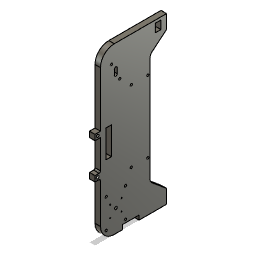
Конвеер Сторона v27 (Autodesk Fusion 360 design; units mm, degrees)
Autodesk Fusion 360 part; units mm, degrees
sketch "Sketch1" plane through (0, 0, 0) normal (1, 0, 0) x (0, 1, 0)
  line L0 (-300, 0) -> (-300, 75)
  line L1 (-275, 100) -> (-25, 100)
  line L2 (0, 75) -> (0, 0)
  arc A0 (-275, 100) -> (-300, 75) centre (-275, 75) ccw
  arc A1 (0, 75) -> (-25, 100) centre (-25, 75) ccw
  line L3 (-300, 0) -> (-300, 25)
  circle A2 centre (-20, 85) radius 5
  circle A3 centre (-280, 85) radius 5
  line L4 (-300, 60) -> (-292, 60)
  line L5 (-292, 60) -> (-292, 30)
  line L6 (-292, 30) -> (-300, 30)
  line L7 (-300, 30) -> (-300, 60)
  line L8 (0, 30) -> (-8, 30)
  line L9 (-8, 30) -> (-8, 60)
  line L10 (-8, 60) -> (0, 60)
  line L11 (0, 60) -> (0, 30)
  line L12 (-275, -20) -> (-300, -20)
  line L13 (-300, -20) -> (-300, 0)
  line L14 (-25, -20) -> (0, -20)
  line L15 (0, -20) -> (0, 0)
  line L16 (-275, -20) -> (-252.9985, 6.4018)
  line L17 (-245.3163, 10) -> (-54.6837, 10)
  line L18 (-47.0015, 6.4018) -> (-25, -20)
  arc A4 (-245.3163, 10) -> (-252.9985, 6.4018) centre (-245.3163, 0) ccw
  arc A5 (-47.0015, 6.4018) -> (-54.6837, 10) centre (-54.6837, 0) ccw
  point P0 (0, 100)
  dimension "d1" = 300
  dimension "d2" = 100
  dimension "d79" = 25
  dimension "d80" = 25
  dimension "d87" = 10
  dimension "d88" = 8
  dimension "d89" = 30
  dimension "d90" = 8
  dimension "d91" = 30
  dimension "d144" = 40
  dimension "d145" = 10
  dimension "d146" = 10
  dimension "d147" = 20
  dimension "d148" = 20
  dimension "d150" = 40
  dimension "d188" = 20
  dimension "d190" = 20
  dimension "d191" = 10
  dimension "d192" = 10
  dimension "d193" = 90
  dimension "d194" = 34.3675
  dimension "d195" = 54.6837
  dimension "d196" = 34.3675
  dimension "d197" = 54.6837
  dimension "d198" = 25
  dimension "d199" = 260
  constraint vertical L0
  constraint horizontal L1
  constraint vertical L2
  constraint coincident L2.end L15.end
  constraint tangent L1 A0
  constraint tangent L0 A0
  constraint coincident P0 L2
  constraint coincident P0 L1
  constraint tangent L2 A1
  constraint tangent L1 A1
  constraint vertical L3
  constraint coincident L0 L3.end
  constraint horizontal L4
  constraint vertical L5
  constraint horizontal L6
  constraint vertical L7
  constraint coincident L0 L4.start
  constraint horizontal L8
  constraint vertical L9
  constraint horizontal L10
  constraint vertical L11
  constraint coincident L2 L8.start
  constraint horizontal L12
  constraint vertical L13
  constraint horizontal L14
  constraint vertical L15
  constraint tangent L16 A4
  constraint tangent L17 A4
  constraint tangent L18 A5
  constraint tangent L17 A5
  measures "d1" distance of L2.end L0.start
  measures "d2" distance of L2.end P0
  measures "d79" radius of A0
  measures "d80" radius of A1
  measures "d87" diameter of A3
  measures "d88" distance of L4.start L4.end
  measures "d89" distance of L4.start L6.end
  measures "d90" distance of L8.start L8.end
  measures "d91" distance of L8.start L10.end
  measures "d144" distance of L1 L10
  measures "d145" vertical distance of A1.centre A2.centre
  measures "d146" diameter of A2
  measures "d147" distance of L2 A2.centre
  measures "d148" distance of L0 A3.centre
  measures "d150" distance of L1 L4
  measures "d188" distance of L0.start L12.end
  measures "d190" distance of L2.end L14.end
  measures "d191" radius of A4
  measures "d192" radius of A5
  measures "d193" distance of L1 L17
  measures "d194" distance of L14.start L18.start
  measures "d195" distance of L2 A5.centre
  measures "d196" distance of L12.start L16.end
  measures "d197" distance of L0 A4.centre
  measures "d198" distance of L12.start L12.end
  measures "d199" distance of A2.centre A3.centre
extrude "Extrude1" add sketch "Sketch1" along normal blind 10 contours L0 L1 L2 A0 A1 L3 L4 L5 L6 L8 L9 L10 L12 L13 L14 L15 L16 L17 L18 A4 A5 | A2 | A3
sketch "Sketch2" plane through (10, 0, 0) normal (1, 0, 0) x (0, 1, 0)
  arc A0 (0, 75) -> (-25, 100) centre (-25, 75) ccw
  line L0 (-25, 100) -> (-275, 100)
  arc A1 (-275, 100) -> (-300, 75) centre (-275, 75) ccw
  line L1 (-300, 75) -> (-300, 60)
  line L2 (0, 60) -> (0, 75)
  line L3 (-8, 30) -> (-8, 60)
  line L4 (-8, 60) -> (0, 60)
  line L5 (-300, 60) -> (-292, 60)
  line L6 (-292, 60) -> (-292, 30)
  line L7 (-292, 30) -> (-300, 30)
  line L8 (-300, 30) -> (-300, -20)
  line L9 (-300, -20) -> (-275, -20)
  line L10 (-275, -20) -> (-252.9985, 6.4018)
  arc A2 (-245.3163, 10) -> (-252.9985, 6.4018) centre (-245.3163, 0) ccw
  line L11 (-245.3163, 10) -> (-54.6837, 10)
  arc A3 (-47.0015, 6.4018) -> (-54.6837, 10) centre (-54.6837, 0) ccw
  line L12 (-47.0015, 6.4018) -> (-25, -20)
  line L13 (-25, -20) -> (0, -20)
  line L14 (0, -20) -> (0, 30)
  line L15 (0, 30) -> (-8, 30)
sketch "Sketch7" plane through (10, 0, 0) normal (1, 0, 0) x (0, 1, 0)
sketch "Sketch8" plane through (10, 0, 0) normal (1, 0, 0) x (0, 1, 0)
sketch "Sketch10" plane through (10, 0, 0) normal (1, 0, 0) x (0, 1, 0)
  line L0 (0, 60) -> (0, 75)
  arc A0 (0, 75) -> (-25, 100) centre (-25, 75) ccw
  line L1 (-25, 100) -> (-275, 100)
  arc A1 (-275, 100) -> (-300, 75) centre (-275, 75) ccw
  line L2 (-300, 75) -> (-300, 60)
  circle A2 centre (-25, 85) radius 5
  circle A3 centre (-275, 85) radius 5
  line L3 (-8, 30) -> (-8, 60)
  line L4 (-8, 60) -> (0, 60)
  line L5 (-300, 60) -> (-292, 60)
  line L6 (-292, 60) -> (-292, 30)
  line L7 (-292, 30) -> (-300, 30)
  line L8 (-300, 30) -> (-300, -20)
  line L9 (-300, -20) -> (-275, -20)
  line L10 (-275, -20) -> (-252.9985, 6.4018)
  arc A4 (-245.3163, 10) -> (-252.9985, 6.4018) centre (-245.3163, 0) ccw
  line L11 (-245.3163, 10) -> (-54.6837, 10)
  arc A5 (-47.0015, 6.4018) -> (-54.6837, 10) centre (-54.6837, 0) ccw
  line L12 (-47.0015, 6.4018) -> (-25, -20)
  line L13 (-25, -20) -> (0, -20)
  line L14 (0, -20) -> (0, 30)
  line L15 (0, 30) -> (-8, 30)
  point P0 (-80, 44)
  dimension "d96" = 10
  dimension "d98" = 10
  dimension "d260" = 25
  dimension "d261" = 25
  dimension "d262" = 25
  dimension "d263" = 25
  measures "d96" diameter of A2
  measures "d98" diameter of A3
  measures "d260" distance of L2 A3.centre
  measures "d261" distance of L0 A2.centre
  measures "d262" distance of A2.centre L4
  measures "d263" distance of A3.centre L5
extrude "Extrude11" cut sketch "Sketch10" against normal blind 100 contours A2 | A3
sketch "Sketch11" plane through (10, 0, 0) normal (1, 0, 0) x (0, 1, 0)
  circle A0 centre (-275, 85) radius 5
  circle A1 centre (-25, 85) radius 5
  line L0 (0, 60) -> (0, 75)
  arc A2 (0, 75) -> (-25, 100) centre (-25, 75) ccw
  line L1 (-25, 100) -> (-275, 100)
  arc A3 (-275, 100) -> (-300, 75) centre (-275, 75) ccw
  line L2 (-300, 75) -> (-300, 60)
  line L3 (-175, 90) -> (-175, 80)
  line L4 (-175, 80) -> (-125, 80)
  line L5 (-175, 80) -> (-125, 80)
  line L6 (-175, 90) -> (-175, 80)
  line L7 (-125, 80) -> (-125, 90)
  line L8 (-125, 90) -> (-175, 90)
  line L9 (-8, 30) -> (-8, 60)
  line L10 (-8, 60) -> (0, 60)
  line L11 (-300, 60) -> (-292, 60)
  line L12 (-292, 60) -> (-292, 30)
  line L13 (-292, 30) -> (-300, 30)
  line L14 (-300, 30) -> (-300, -20)
  line L15 (-300, -20) -> (-275, -20)
  line L16 (-275, -20) -> (-252.9985, 6.4018)
  arc A4 (-245.3163, 10) -> (-252.9985, 6.4018) centre (-245.3163, 0) ccw
  line L17 (-245.3163, 10) -> (-54.6837, 10)
  arc A5 (-47.0015, 6.4018) -> (-54.6837, 10) centre (-54.6837, 0) ccw
  line L18 (-47.0015, 6.4018) -> (-25, -20)
  line L19 (-25, -20) -> (0, -20)
  line L20 (0, -20) -> (0, 30)
  line L21 (0, 30) -> (-8, 30)
  dimension "d174" = 125
  dimension "d175" = 50
  dimension "d176" = 10
  dimension "d259" = 10
  constraint vertical L3
  constraint horizontal L4
  constraint horizontal L5
  constraint vertical L6
  constraint perpendicular L5 L7
  constraint perpendicular L6 L8
  measures "d174" distance of L2 L6
  measures "d175" distance of L3.start L7.end
  measures "d176" distance of L5 L8
  measures "d259" distance of L1 L8
sketch "Sketch12" plane through (10, 0, 0) normal (1, 0, 0) x (0, 1, 0)
  circle A0 centre (-275, 85) radius 5
  circle A1 centre (-25, 85) radius 5
  line L0 (0, 60) -> (0, 75)
  arc A2 (0, 75) -> (-25, 100) centre (-25, 75) ccw
  line L1 (-25, 100) -> (-275, 100)
  arc A3 (-275, 100) -> (-300, 75) centre (-275, 75) ccw
  line L2 (-300, 75) -> (-300, 60)
  line L3 (-275, 85) -> (-260, 85)
  line L4 (-260, 85) -> (-260, 72)
  circle A4 centre (-40, 72) radius 2.5
  circle A5 centre (-260, 72) radius 2.5
  circle A6 centre (-275, 85) radius 2.5
  circle A7 centre (-25, 85) radius 2.5
  line L5 (-8, 30) -> (-8, 60)
  line L6 (-8, 60) -> (0, 60)
  line L7 (-300, 60) -> (-292, 60)
  line L8 (-292, 60) -> (-292, 30)
  line L9 (-292, 30) -> (-300, 30)
  line L10 (-300, 30) -> (-300, -20)
  line L11 (-300, -20) -> (-275, -20)
  line L12 (-275, -20) -> (-252.9985, 6.4018)
  arc A8 (-245.3163, 10) -> (-252.9985, 6.4018) centre (-245.3163, 0) ccw
  line L13 (-245.3163, 10) -> (-54.6837, 10)
  arc A9 (-47.0015, 6.4018) -> (-54.6837, 10) centre (-54.6837, 0) ccw
  line L14 (-47.0015, 6.4018) -> (-25, -20)
  line L15 (-25, -20) -> (0, -20)
  line L16 (0, -20) -> (0, 30)
  line L17 (0, 30) -> (-8, 30)
  dimension "d104" = 13
  dimension "d106" = 5
  dimension "d107" = 5
  dimension "d163" = 5
  dimension "d164" = 5
  dimension "d170" = 15
  dimension "d254" = 28
  dimension "d256" = 40
  dimension "d257" = 10
  dimension "d258" = 15
  constraint coincident A0.centre L3.start
  constraint horizontal L3
  constraint perpendicular L3 L4
  constraint coincident L4.end A5.centre
  constraint concentric A0 A6
  measures "d104" distance of L3.end L4.end
  measures "d106" diameter of A4
  measures "d107" diameter of A5
  measures "d163" diameter of A7
  measures "d164" diameter of A6
  measures "d170" distance of A0.centre L3.end
  measures "d254" distance of L1 A4.centre
  measures "d256" distance of L0 A4.centre
  measures "d257" distance of A2.centre A1.centre
  measures "d258" distance of A2.end A1.centre
extrude "Extrude13" cut sketch "Sketch12" against normal blind 40 contours A4 | A5
extrude "Extrude14" add sketch "Sketch12" against normal blind 10 contours A0 | A1 | A6 | A7
sketch "Sketch13" plane through (0, 0, 100) normal (0, 0, 1) x (-1, 0, 0)
  line L0 (0, 25) -> (0, 275)
  line L1 (0, 275) -> (-10, 275)
  line L2 (-10, 275) -> (-10, 25)
  line L3 (-10, 25) -> (0, 25)
  line L4 (0, 200) -> (-10, 200)
  line L5 (-10, 200) -> (-10, 190)
  line L6 (-10, 190) -> (0, 190)
  line L7 (0, 190) -> (0, 200)
  dimension "d251" = 10
  dimension "d253" = 75
  constraint horizontal L4
  constraint vertical L5
  constraint horizontal L6
  constraint vertical L7
  constraint coincident L2 L5.end
  constraint coincident L0 L4.start
  measures "d251" distance of L4 L6
  measures "d253" distance of L1 L4
extrude "Extrude15" add sketch "Sketch13" along normal blind 10 contours L0 L2 L4 L5 L6 L7
sketch "Sketch14" plane through (10, 0, 0) normal (1, 0, 0) x (0, 1, 0)
  circle A0 centre (-40, 72) radius 2.5
  circle A1 centre (-260, 72) radius 2.5
  line L0 (0, 60) -> (0, 75)
  arc A2 (0, 75) -> (-25, 100) centre (-25, 75) ccw
  line L1 (-25, 100) -> (-190, 100)
  line L2 (-190, 110) -> (-200, 110)
  arc A3 (-275, 100) -> (-300, 75) centre (-275, 75) ccw
  line L3 (-300, 75) -> (-300, 60)
  line L4 (-190, 100) -> (-190, 110)
  circle A4 centre (-195, 105.2223) radius 1.5
  circle A5 centre (-195, 105.2223) radius 2.5
  line L5 (-190, 100) -> (-190, 110)
  line L6 (-200, 110) -> (-200, 100)
  line L7 (-200, 100) -> (-275, 100)
  line L8 (-8, 30) -> (-8, 60)
  line L9 (-8, 60) -> (0, 60)
  line L10 (-300, 60) -> (-292, 60)
  line L11 (-292, 60) -> (-292, 30)
  line L12 (-292, 30) -> (-300, 30)
  line L13 (-300, 30) -> (-300, -20)
  line L14 (-300, -20) -> (-275, -20)
  line L15 (-275, -20) -> (-252.9985, 6.4018)
  arc A6 (-245.3163, 10) -> (-252.9985, 6.4018) centre (-245.3163, 0) ccw
  line L16 (-245.3163, 10) -> (-54.6837, 10)
  arc A7 (-47.0015, 6.4018) -> (-54.6837, 10) centre (-54.6837, 0) ccw
  line L17 (-47.0015, 6.4018) -> (-25, -20)
  line L18 (-25, -20) -> (0, -20)
  line L19 (0, -20) -> (0, 30)
  line L20 (0, 30) -> (-8, 30)
  dimension "d116" = 3
  dimension "d117" = 5
  dimension "d249" = 5
  dimension "d250" = 4.7777
  constraint coincident L2.start L4.end
  constraint perpendicular L2 L4
  constraint concentric A4 A5
  measures "d116" diameter of A4
  measures "d117" diameter of A5
  measures "d249" distance of A4.centre L6
  measures "d250" distance of L2 A4.centre
extrude "Extrude16" cut sketch "Sketch14" against normal blind 13 contours A4 | A5
thread "Thread6" "ISO Metric profile 5.0 M5x0.8 6H" major diameter 5.12 minor diameter 4.234 pitch 0.8 angle 60 resizes the face on face at (6.6667, -194.2038, 107.5921)
sketch "Sketch15" plane through (10, 0, 0) normal (1, 0, 0) x (0, 1, 0)
  circle A0 centre (-195, 105.2223) radius 2.117
  circle A1 centre (-40, 72) radius 2.5
  circle A2 centre (-260, 72) radius 2.5
  line L0 (0, 60) -> (0, 75)
  arc A3 (0, 75) -> (-25, 100) centre (-25, 75) ccw
  line L1 (-25, 100) -> (-190, 100)
  line L2 (-190, 110) -> (-200, 110)
  arc A4 (-275, 100) -> (-300, 75) centre (-275, 75) ccw
  line L3 (-300, 75) -> (-300, 60)
  circle A5 centre (-195, 105.2223) radius 3
  line L4 (-190, 100) -> (-190, 110)
  line L5 (-200, 110) -> (-200, 100)
  line L6 (-200, 100) -> (-275, 100)
  line L7 (-8, 30) -> (-8, 60)
  line L8 (-8, 60) -> (0, 60)
  line L9 (-300, 60) -> (-292, 60)
  line L10 (-292, 60) -> (-292, 30)
  line L11 (-292, 30) -> (-300, 30)
  line L12 (-300, 30) -> (-300, -20)
  line L13 (-300, -20) -> (-275, -20)
  line L14 (-275, -20) -> (-252.9985, 6.4018)
  arc A6 (-245.3163, 10) -> (-252.9985, 6.4018) centre (-245.3163, 0) ccw
  line L15 (-245.3163, 10) -> (-54.6837, 10)
  arc A7 (-47.0015, 6.4018) -> (-54.6837, 10) centre (-54.6837, 0) ccw
  line L16 (-47.0015, 6.4018) -> (-25, -20)
  line L17 (-25, -20) -> (0, -20)
  line L18 (0, -20) -> (0, 30)
  line L19 (0, 30) -> (-8, 30)
  dimension "d120" = 6
  constraint concentric A0 A5
  measures "d120" diameter of A5
extrude "Extrude17" cut sketch "Sketch15" against normal blind 16.5 contours A5
thread "Thread7" "ISO Metric profile 6.0 M6x1 6H" major diameter 6.147 minor diameter 5.035 pitch 1 angle 60 resizes the face on face at (6.6667, -192.9053, 107.3699)
fillet "Fillet2" radius 2.5 2 edges at (5, -200, 100) (5, -190, 100)
sketch "Sketch16" plane through (10, 0, 0) normal (1, 0, 0) x (0, 1, 0)
  line L0 (-270.5, 61.5) -> (-249.5, 61.5)
  line L1 (-249.5, 61.5) -> (-249.5, 82.5)
  line L2 (-249.5, 82.5) -> (-270.5, 82.5)
  line L3 (-270.5, 82.5) -> (-270.5, 61.5)
  line L4 (-270.5, 61.5) -> (-249.5, 82.5) construction
  line L5 (-249.5, 61.5) -> (-270.5, 82.5) construction
  circle A0 centre (-270.5, 82.5) radius 1
  circle A1 centre (-249.5, 82.5) radius 1
  circle A2 centre (-249.5, 61.5) radius 1
  circle A3 centre (-270.5, 61.5) radius 1
  line L6 (-290, 93) -> (-230, 93)
  line L7 (-230, 93) -> (-230, 51)
  line L8 (-230, 51) -> (-290, 51)
  line L9 (-290, 51) -> (-290, 93)
  line L10 (-290, 93) -> (-230, 51) construction
  line L11 (-230, 93) -> (-290, 51) construction
  line L12 (-260, 72) -> (-245.6634, 92.4808)
  line L13 (-260, 72) -> (-260, 89.5)
  line L14 (-260, 89.5) -> (-233.5, 89.5)
  line L15 (-233.5, 89.5) -> (-286.5, 89.5)
  line L16 (-260, 72) -> (-260, 54.5)
  circle A4 centre (-286.5, 89.5) radius 2
  circle A5 centre (-233.5, 89.5) radius 2
  line L17 (-260, 54.5) -> (-286.5, 54.5)
  line L18 (-286.5, 54.5) -> (-233.5, 54.5)
  circle A6 centre (-286.5, 54.5) radius 2
  circle A7 centre (-233.5, 54.5) radius 2
  point P0 (-260, 72)
  point P1 (-260, 72)
  point P2 (-260, 72)
  dimension "d127" = 21
  dimension "d128" = 21
  dimension "d129" = 2
  dimension "d130" = 2
  dimension "d131" = 2
  dimension "d132" = 2
  dimension "d133" = 60
  dimension "d134" = 42
  dimension "d135" = 25
  dimension "d165" = 17.5
  dimension "d166" = 26.5
  dimension "d167" = 53
  dimension "d168" = 17.5
  dimension "d179" = 4
  dimension "d180" = 4
  dimension "d181" = 53
  dimension "d182" = 4
  dimension "d183" = 4
  dimension "d184" = 26.5
  constraint horizontal L0
  constraint perpendicular L0 L1
  constraint parallel L0 L2
  constraint parallel L1 L3
  constraint coincident L4 P2
  constraint coincident L5 P2
  constraint coincident L2.end L3.start
  constraint coincident L1.end L2.start
  constraint coincident L0.end L1.start
  constraint coincident L0.start L3.end
  constraint horizontal L6
  constraint perpendicular L6 L7
  constraint parallel L6 L8
  constraint parallel L7 L9
  constraint coincident L10 P2
  constraint coincident L11 P2
  constraint coincident P2 P1
  constraint perpendicular L10 L12
  constraint perpendicular L2 L13
  constraint perpendicular L13 L14
  constraint perpendicular L13 L15
  constraint perpendicular L0 L16
  constraint coincident L15.end A4.centre
  constraint coincident L14.end L15.start
  constraint perpendicular L16 L17
  constraint perpendicular L16 L18
  constraint coincident L17.end L18.start
  constraint coincident L18.end A7.centre
  measures "d127" distance of L1.end L2.end
  measures "d128" distance of L0.end L1.end
  measures "d129" diameter of A0
  measures "d130" diameter of A1
  measures "d131" diameter of A2
  measures "d132" diameter of A3
  measures "d133" distance of L7.end L8.end
  measures "d134" distance of L6.end L7.end
  measures "d135" distance of P2 L12.end
  measures "d165" distance of P2 L13.end
  measures "d166" distance of L13.end L14.end
  measures "d167" distance of L14.end L15.end
  measures "d168" distance of P2 L16.end
  measures "d179" diameter of A4
  measures "d180" diameter of A5
  measures "d181" distance of L17.end L18.end
  measures "d182" diameter of A6
  measures "d183" diameter of A7
  measures "d184" distance of L16 L17.end
extrude "Extrude23" cut sketch "Sketch11" against normal blind 60 contours L3 L4 L5 L6 L7 L8
extrude "Extrude19" cut sketch "Sketch16" against normal blind 45 contours L0 L3 A3 | L0 L3 A3 | L2 L3 A0 | L2 L3 A0 | L0 L1 A2 | L0 L1 A2 | L1 L2 A1 | L1 L2 A1 | A4 | A5 | A6 | A7
sketch "Sketch18" plane through (10, 0, 0) normal (1, 0, 0) x (0, 1, 0)
  line L0 (-20, -9.7401) -> (-5, -9.7401)
  line L1 (-5, -9.7401) -> (-5, 0.2599)
  line L2 (-5, 0.2599) -> (-20, 0.2599)
  line L3 (-20, 0.2599) -> (-20, -9.7401)
  dimension "d155" = 10
  dimension "d200" = 15
  dimension "d247" = 5
  dimension "d248" = 0.2599
  constraint horizontal L0
  constraint vertical L1
  constraint horizontal L2
  constraint vertical L3
  measures "d155" distance of L0.end L1.end
  measures "d200" distance of L1.end L2.end
  measures "d247" distance of origin L1
  measures "d248" distance of origin L2
extrude "Extrude21" cut sketch "Sketch18" against normal blind 41
sketch "Sketch19" plane through (10, 0, 0) normal (1, 0, 0) x (0, 1, 0)
  line L0 (-135, 100) -> (-125, 100)
  line L1 (-125, 100) -> (-125, 110)
  line L2 (-125, 110) -> (-135, 110)
  line L3 (-135, 110) -> (-135, 100)
  circle A0 centre (-130, 105) radius 2.5
  dimension "d156" = 10
  dimension "d157" = 10
  dimension "d158" = 5
  dimension "d243" = 5
  dimension "d244" = 5
  dimension "d245" = 125
  dimension "d246" = 110
  constraint horizontal L0
  constraint vertical L1
  constraint horizontal L2
  constraint vertical L3
  measures "d156" distance of L1 L3
  measures "d157" distance of L0 L2
  measures "d158" diameter of A0
  measures "d243" distance of L0 A0.centre
  measures "d244" distance of L1 A0.centre
  measures "d245" distance of origin L1
  measures "d246" distance of origin L2
extrude "Extrude22" add sketch "Sketch19" against normal blind 10
sketch "Sketch20" plane through (10, 0, 0) normal (1, 0, 0) x (0, 1, 0)
  circle A0 centre (-130, 105) radius 2.5
  line L0 (-5, -9.7401) -> (-20, -9.7401)
  line L1 (-20, -9.7401) -> (-20, 0.2599)
  line L2 (-20, 0.2599) -> (-5, 0.2599)
  line L3 (-5, 0.2599) -> (-5, -9.7401)
  circle A1 centre (-233.5, 54.5) radius 2
  circle A2 centre (-249.5, 82.5) radius 1
  circle A3 centre (-249.5, 61.5) radius 1
  circle A4 centre (-286.5, 54.5) radius 2
  circle A5 centre (-233.5, 89.5) radius 2
  circle A6 centre (-270.5, 82.5) radius 1
  circle A7 centre (-270.5, 61.5) radius 1
  circle A8 centre (-286.5, 89.5) radius 2
  line L4 (-175, 80) -> (-175, 90)
  line L5 (-175, 90) -> (-125, 90)
  line L6 (-125, 90) -> (-125, 80)
  line L7 (-125, 80) -> (-175, 80)
  circle A9 centre (-195, 105.2223) radius 2.5175
  circle A10 centre (-40, 72) radius 2.5
  circle A11 centre (-260, 72) radius 2.5
  line L8 (0, 60) -> (0, 75)
  arc A12 (0, 75) -> (-25, 100) centre (-25, 75) ccw
  line L9 (-25, 100) -> (-125, 100)
  line L10 (-125, 100) -> (-125, 110)
  line L11 (-125, 110) -> (-135, 110)
  line L12 (-135, 110) -> (-135, 100)
  arc A13 (-190, 102.5) -> (-187.5, 100) centre (-187.5, 102.5) ccw
  line L13 (-190, 102.5) -> (-190, 110)
  line L14 (-190, 110) -> (-200, 110)
  line L15 (-200, 110) -> (-200, 102.5)
  arc A14 (-202.5, 100) -> (-200, 102.5) centre (-202.5, 102.5) ccw
  line L16 (-202.5, 100) -> (-275, 100)
  arc A15 (-275, 100) -> (-300, 75) centre (-275, 75) ccw
  line L17 (-300, 75) -> (-300, 60)
  line L18 (-40, 72) -> (-50, 72)
  line L19 (-50, 74.5) -> (-40, 74.5)
  line L20 (-40, 69.5) -> (-50, 69.5)
  arc A16 (-50, 74.5) -> (-50, 69.5) centre (-50, 72) ccw
  line L21 (-300, 60) -> (-292, 60)
  line L22 (-292, 60) -> (-292, 30)
  line L23 (-292, 30) -> (-300, 30)
  line L24 (-300, 30) -> (-300, -20)
  line L25 (-300, -20) -> (-275, -20)
  line L26 (-275, -20) -> (-252.9985, 6.4018)
  arc A17 (-245.3163, 10) -> (-252.9985, 6.4018) centre (-245.3163, 0) ccw
  line L27 (-245.3163, 10) -> (-54.6837, 10)
  arc A18 (-47.0015, 6.4018) -> (-54.6837, 10) centre (-54.6837, 0) ccw
  line L28 (-47.0015, 6.4018) -> (-25, -20)
  line L29 (-25, -20) -> (0, -20)
  line L30 (-8, 30) -> (-8, 60)
  line L31 (-8, 60) -> (0, 60)
  line L32 (-135, 100) -> (-187.5, 100)
  line L33 (0, -20) -> (0, 30)
  line L34 (0, 30) -> (-8, 30)
  dimension "d185" = 5
  dimension "d240" = 10
  dimension "d242" = 10
  constraint coincident A10.centre L18.start
  constraint horizontal L18
  constraint coincident L18.end A16.centre
  constraint coincident L19.start A16
  constraint coincident A10 L19.end
  constraint tangent A10 L19
  constraint coincident A10 L20.start
  constraint tangent L20 A16
  constraint parallel L9 L20
  constraint coincident L19 A16.start
  measures "d185" diameter of A16
  measures "d240" horizontal distance of L19.start L19.end
  measures "d242" distance of A10.centre L18.end
extrude "Extrude24" cut sketch "Sketch20" against normal blind 35 contours A10 L19 L20 A16
sketch "Sketch21" plane through (10, 0, 0) normal (1, 0, 0) x (0, 1, 0)
  circle A0 centre (-260, 72) radius 2.5
  line L0 (-40, 69.5) -> (-50, 69.5)
  arc A1 (-50, 74.5) -> (-50, 69.5) centre (-50, 72) ccw
  line L1 (-50, 74.5) -> (-40, 74.5)
  arc A2 (-40, 69.5) -> (-40, 74.5) centre (-40, 72) ccw
  circle A3 centre (-195, 105.2223) radius 2.5175
  line L2 (0, 60) -> (0, 75)
  arc A4 (0, 75) -> (-25, 100) centre (-25, 75) ccw
  line L3 (-25, 100) -> (-125, 100)
  line L4 (-125, 100) -> (-125, 110)
  line L5 (-125, 110) -> (-135, 110)
  line L6 (-135, 110) -> (-135, 100)
  arc A5 (-190, 102.5) -> (-187.5, 100) centre (-187.5, 102.5) ccw
  line L7 (-190, 102.5) -> (-190, 110)
  line L8 (-190, 110) -> (-200, 110)
  line L9 (-200, 110) -> (-200, 102.5)
  arc A6 (-202.5, 100) -> (-200, 102.5) centre (-202.5, 102.5) ccw
  line L10 (-202.5, 100) -> (-275, 100)
  arc A7 (-275, 100) -> (-300, 75) centre (-275, 75) ccw
  line L11 (-300, 75) -> (-300, 60)
  line L12 (-300, 60) -> (-292, 60)
  line L13 (-292, 60) -> (-292, 30)
  line L14 (-292, 30) -> (-300, 30)
  line L15 (-300, 30) -> (-300, -20)
  line L16 (-300, -20) -> (-275, -20)
  line L17 (-275, -20) -> (-252.9985, 6.4018)
  arc A8 (-245.3163, 10) -> (-252.9985, 6.4018) centre (-245.3163, 0) ccw
  line L18 (-245.3163, 10) -> (-54.6837, 10)
  arc A9 (-47.0015, 6.4018) -> (-54.6837, 10) centre (-54.6837, 0) ccw
  line L19 (-47.0015, 6.4018) -> (-25, -20)
  line L20 (-25, -20) -> (0, -20)
  line L21 (-175, 80) -> (-175, 90)
  line L22 (-175, 90) -> (-125, 90)
  line L23 (-125, 90) -> (-125, 80)
  line L24 (-125, 80) -> (-175, 80)
  circle A10 centre (-286.5, 89.5) radius 2
  circle A11 centre (-270.5, 61.5) radius 1
  circle A12 centre (-270.5, 82.5) radius 1
  circle A13 centre (-233.5, 89.5) radius 2
  circle A14 centre (-286.5, 54.5) radius 2
  circle A15 centre (-249.5, 61.5) radius 1
  circle A16 centre (-249.5, 82.5) radius 1
  circle A17 centre (-233.5, 54.5) radius 2
  line L25 (-5, -9.7401) -> (-20, -9.7401)
  line L26 (-20, -9.7401) -> (-20, 0.2599)
  line L27 (-20, 0.2599) -> (-5, 0.2599)
  line L28 (-5, 0.2599) -> (-5, -9.7401)
  circle A18 centre (-130, 105) radius 2.5
  circle A19 centre (-80, 44) radius 2
  circle A20 centre (-80, 14) radius 2
  circle A21 centre (-210, 44) radius 2
  circle A22 centre (-210, 14) radius 2
  line L29 (-8, 30) -> (-8, 60)
  line L30 (-8, 60) -> (0, 60)
  line L31 (-135, 100) -> (-187.5, 100)
  line L32 (0, -20) -> (0, 30)
  line L33 (0, 30) -> (-8, 30)
  dimension "d211" = 4
  dimension "d212" = 4
  dimension "d214" = 4
  dimension "d215" = 4
  dimension "d232" = 30
  dimension "d233" = 130
  dimension "d234" = 30
  dimension "d235" = 4
  dimension "d236" = 90
  dimension "d237" = 4
  dimension "d238" = 80
  dimension "d239" = 82
  measures "d211" diameter of A19
  measures "d212" diameter of A20
  measures "d214" diameter of A21
  measures "d215" diameter of A22
  measures "d232" distance of A19.centre A20.centre
  measures "d233" distance of A20.centre A22.centre
  measures "d234" distance of A21.centre A22.centre
  measures "d235" distance of L18 A22.centre
  measures "d236" distance of L15 A22.centre
  measures "d237" distance of L18 A20.centre
  measures "d238" distance of L2 A19.centre
  measures "d239" distance of L13 A21.centre
extrude "Extrude25" cut sketch "Sketch21" against normal blind 35 contours A19 | A20 | A21 | A22
sketch "Sketch22" plane through (10, 0, 0) normal (1, 0, 0) x (0, 1, 0)
  circle A0 centre (-210, 14) radius 2
  circle A1 centre (-80, 44) radius 2
  circle A2 centre (-210, 44) radius 2
  circle A3 centre (-80, 14) radius 2
  circle A4 centre (-260, 72) radius 2.5
  line L0 (-40, 69.5) -> (-50, 69.5)
  arc A5 (-50, 74.5) -> (-50, 69.5) centre (-50, 72) ccw
  line L1 (-50, 74.5) -> (-40, 74.5)
  arc A6 (-40, 69.5) -> (-40, 74.5) centre (-40, 72) ccw
  circle A7 centre (-195, 105.2223) radius 2.5175
  line L2 (0, 60) -> (0, 75)
  arc A8 (0, 75) -> (-25, 100) centre (-25, 75) ccw
  line L3 (-25, 100) -> (-125, 100)
  line L4 (-125, 100) -> (-125, 110)
  line L5 (-125, 110) -> (-135, 110)
  line L6 (-135, 110) -> (-135, 100)
  arc A9 (-190, 102.5) -> (-187.5, 100) centre (-187.5, 102.5) ccw
  line L7 (-190, 102.5) -> (-190, 110)
  line L8 (-190, 110) -> (-200, 110)
  line L9 (-200, 110) -> (-200, 102.5)
  arc A10 (-202.5, 100) -> (-200, 102.5) centre (-202.5, 102.5) ccw
  line L10 (-202.5, 100) -> (-275, 100)
  arc A11 (-275, 100) -> (-300, 75) centre (-275, 75) ccw
  line L11 (-300, 75) -> (-300, 60)
  line L12 (-300, 60) -> (-292, 60)
  line L13 (-292, 60) -> (-292, 30)
  line L14 (-292, 30) -> (-300, 30)
  line L15 (-300, 30) -> (-300, -20)
  line L16 (-300, -20) -> (-275, -20)
  line L17 (-275, -20) -> (-252.9985, 6.4018)
  arc A12 (-245.3163, 10) -> (-252.9985, 6.4018) centre (-245.3163, 0) ccw
  line L18 (-245.3163, 10) -> (-54.6837, 10)
  arc A13 (-47.0015, 6.4018) -> (-54.6837, 10) centre (-54.6837, 0) ccw
  line L19 (-47.0015, 6.4018) -> (-25, -20)
  line L20 (-25, -20) -> (0, -20)
  line L21 (-175, 80) -> (-175, 90)
  line L22 (-175, 90) -> (-125, 90)
  line L23 (-125, 90) -> (-125, 80)
  line L24 (-125, 80) -> (-175, 80)
  circle A14 centre (-286.5, 89.5) radius 2
  circle A15 centre (-270.5, 61.5) radius 1
  circle A16 centre (-270.5, 82.5) radius 1
  circle A17 centre (-233.5, 89.5) radius 2
  circle A18 centre (-286.5, 54.5) radius 2
  circle A19 centre (-249.5, 61.5) radius 1
  circle A20 centre (-249.5, 82.5) radius 1
  circle A21 centre (-233.5, 54.5) radius 2
  line L25 (-5, -9.7401) -> (-20, -9.7401)
  line L26 (-20, -9.7401) -> (-20, 0.2599)
  line L27 (-20, 0.2599) -> (-5, 0.2599)
  line L28 (-5, 0.2599) -> (-5, -9.7401)
  circle A22 centre (-130, 105) radius 2.5
  line L29 (-65, 60) -> (-25, 60)
  line L30 (-25, 60) -> (-25, 85)
  line L31 (-25, 85) -> (-65, 85)
  line L32 (-65, 85) -> (-65, 60)
  circle A23 centre (-60, 65) radius 2
  circle A24 centre (-30, 80) radius 2
  line L33 (-8, 30) -> (-8, 60)
  line L34 (-8, 60) -> (0, 60)
  line L35 (-135, 100) -> (-187.5, 100)
  line L36 (0, -20) -> (0, 30)
  line L37 (0, 30) -> (-8, 30)
  dimension "d218" = 40
  dimension "d219" = 25
  dimension "d220" = 4
  dimension "d222" = 4
  dimension "d223" = 25
  dimension "d224" = 15
  dimension "d225" = 5
  dimension "d226" = 35
  dimension "d227" = 35
  dimension "d229" = 5
  constraint horizontal L29
  constraint vertical L30
  constraint horizontal L31
  constraint vertical L32
  measures "d218" distance of L29.start L29.end
  measures "d219" distance of L29.start L31.end
  measures "d220" diameter of A23
  measures "d222" diameter of A24
  measures "d223" distance of L2 L30
  measures "d224" distance of L3 L31
  measures "d225" distance of L29 A23.centre
  measures "d226" distance of L30 A23.centre
  measures "d227" distance of L32 A24.centre
  measures "d229" distance of L31 A24.centre
extrude "Extrude26" cut sketch "Sketch22" against normal blind 120 contours A23 | A24
extrude "Extrude27" add 1 faces at (3.3333, -2.6667, 30) along direction (0, 0, 1) blind 30
